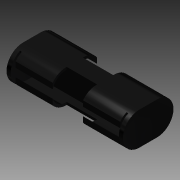
# Autodesk Inventor part: Battery Pack
Saved by Autodesk Inventor 2014 (Build 180170000, 170)
## iProperties
Created: 2014-03-06
Part Number: Battery Pack
Material: Generic
Document SubType Name: Modeling
Designer: Alex
Density: 1 g/cm^3
Appearance: Glossy - Black
Author: Alex
Autodesk Inventor part; units mm, degrees
note: some values were not read from the file. Chosen so that the rebuilt part matches the saved one: sketch regions of "Extrusion2".
ref_plane "YZ Plane" through (0, 0, 0) normal (1, 0, 0) x (0, 1, 0)
sketch "Sketch1" plane through (0, 0, 0) normal (0, 0, 1) x (1, 0, 0)
  line L0 (0, 0) -> (58.42, 0)
  line L1 (58.42, 0) -> (58.42, 16.51)
  line L2 (58.42, 16.51) -> (0, 16.51)
  line L3 (0, 16.51) -> (0, 0)
  dimension "d0" = 16.51
  dimension "d1" = 58.42
  constraints: 8 end point, 2 parallel, 1 horizontal, 1 perpendicular
  measures "d0" distance of L2.end L0.start
  measures "d1" distance of L1.end L2.end
extrude "Extrusion1" add sketch "Sketch1" along normal blind 25.4
fillet "Fillet1" radius 8.255 4 edges at (29.21, 16.51, 25.4) (29.21, 0, 25.4) (29.21, 16.51, 0) (29.21, 0, 0)
ref_plane "Work Plane1" through (56.388, 8.255, 8.255) normal (1, 0, 0) x (0, 0, -1)
sketch "Sketch2" plane through (56.388, 8.255, 8.255) normal (1, 0, 0) x (0, 0, -1)
  arc A0 (0, -8.255) -> (0, 8.255) centre (0, 0) ccw projected
  line L0 (0, 8.255) -> (-8.89, 8.255) projected
  arc A1 (-8.89, 8.255) -> (-8.89, -8.255) centre (-8.89, 0) ccw projected
  line L1 (0, -8.255) -> (-8.89, -8.255) projected
  arc A2 (0, -6.985) -> (0, 6.985) centre (0, 0) ccw
  arc A3 (-8.89, 6.985) -> (-8.89, -6.985) centre (-8.89, 0) ccw
  line L2 (0, 6.985) -> (-8.89, 6.985)
  line L3 (0, -6.985) -> (-8.89, -6.985)
  line L4 (-4.953, 6.985) -> (-3.937, 6.985)
  line L5 (-3.937, 6.985) -> (-3.937, -6.985)
  line L6 (-3.937, -6.985) -> (-4.953, -6.985)
  line L7 (-4.953, -6.985) -> (-4.953, 6.985)
  line L8 (-8.89, 0) -> (-4.953, 0) construction
  line L9 (-3.937, 0) -> (0, 0) construction
  point P0 (8.255, -8.255)
  dimension "d6" = 1.27
  dimension "d7" = 1.27
  dimension "d9" = 1.016
  constraints: 16 end point, 4 point on circle, 4 tangent, 2 centre point, 2 coincident, 2 midpoint, 2 parallel, 2 point on line, 1 collinear, 1 horizontal, 1 perpendicular
  measures "d6" radial gap between concentric circles of A0 A2
  measures "d7" radial gap between concentric circles of A1 A3
  measures "d9" distance between parallel lines of L5 L7
ref_plane "Work Plane2" through (2.032, 8.255, 8.255) normal (-1, 0, 0) x (0, 0, 1)
extrude "Extrusion2" cut sketch "Sketch2" against normal up to surface (54.356 mm away) contours L3 L5 L2 A2 | L3 A3 L2 L7
sketch "Sketch3" plane through (0, 16.51, 8.255) normal (0, 1, 0) x (1, 0, 0)
  line L0 (0, 0) -> (58.42, 0) construction
  line L1 (0, 0) -> (0, 0) construction
  line L2 (0, 0) -> (58.42, 0) construction
  line L3 (58.42, 0) -> (58.42, 0) construction
  line L4 (58.42, 0) -> (0, 0) construction
  line L5 (0, -8.89) -> (0, -8.89) construction
  line L6 (0, -8.89) -> (58.42, -8.89) construction
  line L7 (58.42, -8.89) -> (58.42, -8.89) construction
  line L8 (58.42, -8.89) -> (0, -8.89) construction
  line L9 (21.59, -8.509) -> (36.83, -8.509)
  line L10 (36.83, -0.381) -> (21.59, -0.381)
  line L11 (58.42, -8.89) -> (58.42, -17.145) construction
  line L12 (21.59, -0.381) -> (21.59, 6.6675)
  line L13 (36.83, -0.381) -> (36.83, 6.6675)
  line L14 (36.83, -8.509) -> (36.83, -15.5575)
  line L15 (21.59, -8.509) -> (21.59, -15.5575)
  line L16 (2.921, -15.5575) -> (21.59, -15.5575)
  line L17 (36.83, -15.5575) -> (55.499, -15.5575)
  line L18 (55.499, 6.6675) -> (36.83, 6.6675)
  line L19 (21.59, 6.6675) -> (2.921, 6.6675)
  line L20 (2.921, 3.4925) -> (2.032, 3.4925)
  line L21 (2.032, 3.4925) -> (2.032, -12.3825)
  line L22 (2.032, -12.3825) -> (2.921, -12.3825)
  line L23 (2.921, 6.6675) -> (2.921, 3.4925)
  line L24 (2.921, -12.3825) -> (2.921, -15.5575)
  line L25 (55.499, 3.4925) -> (56.388, 3.4925)
  line L26 (56.388, 3.4925) -> (56.388, -12.3825)
  line L27 (56.388, -12.3825) -> (55.499, -12.3825)
  line L28 (55.499, -15.5575) -> (55.499, -12.3825)
  line L29 (55.499, 3.4925) -> (55.499, 6.6675)
  line L30 (2.032, -22.225) -> (2.032, 13.335) projected
  line L31 (2.032, 3.4925) -> (2.032, 8.255)
  line L32 (2.032, 8.255) -> (56.388, 8.255)
  line L33 (56.388, 8.255) -> (56.388, 3.4925)
  line L34 (2.032, -12.3825) -> (2.032, -17.145)
  line L35 (2.032, -17.145) -> (56.388, -17.145)
  line L36 (56.388, -17.145) -> (56.388, -12.3825)
  line L37 (58.42, 0) -> (58.42, -8.89) projected
  point P0 (0, 8.255)
  point P1 (2.032, -10.5301)
  dimension "d12" = 8.128
  dimension "d21" = 22.225
  dimension "d23" = 15.24
  dimension "d25" = 15.24
  dimension "d27" = 22.225
  dimension "d49" = 2.032
  dimension "d50" = 2.032
  dimension "d51" = 0.381
  dimension "d52" = 7.0485
  dimension "d53" = 7.0485
  dimension "d54" = 7.0485
  dimension "d55" = 7.0485
  dimension "d56" = 0.889
  dimension "d57" = 0.889
  dimension "d58" = 0.889
  dimension "d59" = 0.889
  dimension "d60" = 15.875
  dimension "d61" = 15.875
  dimension "d62" = 18.669
  dimension "d63" = 18.669
  dimension "d64" = 18.669
  dimension "d65" = 18.669
  dimension "d66" = 3.175
  dimension "d67" = 3.175
  dimension "d68" = 3.175
  dimension "d69" = 3.175
  dimension "d70" = 1.5875
  dimension "d71" = 1.5875
  constraints: 52 end point, 15 perpendicular, 12 parallel, 5 horizontal, 3 vertical, 1 collinear, 1 horizontal alignment, 1 point on line
  measures "d12" distance between parallel lines of L10 L9
  measures "d21" distance between parallel lines of L16 L19
  measures "d23" distance between parallel lines of L13 L12
  measures "d25" distance between parallel lines of L14 L15
  measures "d27" distance between parallel lines of L18 L17
  measures "d49" distance from line of point (0, 8.255) L31
  measures "d50" distance between parallel lines of L37 L33
  measures "d51" distance between parallel lines of L0 L10
  measures "d52" distance between parallel lines of L19 L10
  measures "d53" distance between parallel lines of L16 L9
  measures "d54" distance between parallel lines of L10 L18
  measures "d55" distance between parallel lines of L9 L17
  measures "d56" distance of L21.end L22.end
  measures "d57" distance of L20.start L20.end
  measures "d58" distance of L25.start L25.end
  measures "d59" distance of L26.end L27.end
  measures "d60" distance between parallel lines of L27 L25
  measures "d61" distance between parallel lines of L22 L20
  measures "d62" distance between parallel lines of L15 L24
  measures "d63" distance of L12.end L19.end
  measures "d64" distance of L18.start L13.end
  measures "d65" distance of L14.end L17.end
  measures "d66" distance between parallel lines of L19 L20
  measures "d67" distance between parallel lines of L22 L16
  measures "d68" distance between parallel lines of L18 L25
  measures "d69" distance between parallel lines of L17 L27
  measures "d70" distance between parallel lines of L19 L32
  measures "d71" distance between parallel lines of L35 L16
extrude "Extrusion3" cut sketch "Sketch3" against normal through all contours L9 L14 L17 L28 L27 L36 L35 L30 L22 L24 L16 L15 | L30 L32 L33 L25 L29 L18 L13 L10 L12 L19 L23 L20
equation "\"d25\" = d23"
equation "\"d27\" = d21"
equation "\"d50\" = d49"
equation "\"d52\" = d53"
equation "\"d54\" = d52"
equation "\"d57\" = d56"
equation "\"d58\" = d56"
equation "\"d59\" = d56"
equation "\"d62\" = d65"
equation "\"d63\" = d64"
equation "\"d66\" = d67"
equation "\"d68\" = d69"
equation "\"d70\" = d71"
equation "\"d19\" = d18"
equation "\"d26\" = d24"
equation "\"d18\" = 2.921"
equation "\"d24\" = 18.669"
body "Solid1"
